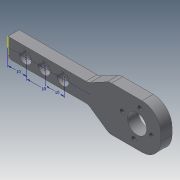
# Autodesk Inventor part: Xmovementarm
Saved by Autodesk Inventor 2019 (Build 230136000, 136)
## iProperties
Created: 2019-01-13
Part Number: Xmovementarm
Material: Aluminum 6061
Document SubType Name: Modeling
Designer: LillaHunden
Density: 2.7 g/cm^3
Appearance: Aluminum - Flat
Mass: 17.0465 g
Surface Area: 40.0048 cm^2
Volume: 6.31351 cm^3
Author: LillaHunden
Autodesk Inventor part; units mm, degrees
ref_plane "YZ Plane" through (0, 0, 0) normal (1, 0, 0) x (0, 1, 0)
ref_plane "XZ Plane" through (0, 0, 0) normal (0, 1, 0) x (-1, 0, 0)
ref_plane "XY Plane" through (0, 0, 0) normal (0, 0, 1) x (1, 0, 0)
sketch "Sketch1" plane through (0, 0, 0) normal (0, 0, 1) x (1, 0, 0)
  line L0 (86.0355, 15.9499) -> (58.5676, 15.9499)
  line L1 (58.5676, 15.9499) -> (58.5676, -7.7845)
  line L2 (58.5676, -7.7845) -> (86.0355, -7.7845)
  line L3 (86.0355, -7.7845) -> (86.0355, 15.9499)
  line L4 (6.25, 0) -> (40, 0) projected
  line L5 (40, 0) -> (40, 10) projected
  line L6 (4.75, 10) -> (40, 10) projected
  line L7 (40, 10) -> (58.5676, 10)
  line L8 (40, 0) -> (58.5676, 0)
  line L9 (58.5676, 15.9499) -> (47.3956, 10)
  line L10 (58.5676, -7.7845) -> (47.3956, 0)
  circle A0 centre (34, 5) radius 2 projected
  line L11 (4.75, 10) -> (4.75, 1.5) projected
  circle A1 centre (14, 5) radius 1.5 projected
  circle A2 centre (34, 5) radius 1.5 projected
  circle A3 centre (24, 5) radius 1.5 projected
  line L12 (6.25, 0) -> (4.75, 1.5) projected
  constraints: 16 end point, 4 point on line, 3 perpendicular, 2 parallel, 1 horizontal
extrude "Extrusion1" add sketch "Sketch1" along normal blind 6 contours L3 L2 L1 L0 | L1 L7 L9 | L1 L8 L5 L7 | L10 L8 L1 | L5 L4 L12 L11 L6 | A0 | A1 | A2 | A3
sketch "Sketch2" plane through (0, 0, 0) normal (0, 0, -1) x (-1, 0, 0)
  circle A0 centre (-73.4131, 4.0423) radius 11 construction
  spline S0 degree 3 poles (-70.2716, -3.9978) (-70.3138, -4.1848) (-70.3928, -4.3613) (-70.5018, -4.5192) (-70.5089, -4.5295) (-70.5162, -4.5398) (-70.5235, -4.5499) (-70.6171, -4.6787) (-70.7297, -4.7921) (-70.8576, -4.8849) (-70.8752, -4.8977) (-70.8931, -4.9101) (-70.9114, -4.9221) (-70.9198, -4.9276) (-70.9284, -4.9331) (-70.9369, -4.9385) (-71.0158, -4.988) (-71.099, -5.0293) (-71.1859, -5.0613) (-71.2374, -5.0803) (-71.2903, -5.096) (-71.3441, -5.1084) (-71.3753, -5.1156) (-71.4068, -5.1217) (-71.4386, -5.1267) (-71.5837, -5.1495) (-71.732, -5.1491) (-71.8775, -5.1259) (-71.8956, -5.123) (-71.9137, -5.1198) (-71.9318, -5.1161) (-71.9426, -5.114) (-71.9535, -5.1117) (-71.9643, -5.1092) (-72.0615, -5.0873) (-72.1559, -5.0551) (-72.2453, -5.0124) (-72.3176, -4.9779) (-72.3864, -4.9368) (-72.4503, -4.8889) (-72.4664, -4.8768) (-72.4822, -4.8643) (-72.4968, -4.8497) knots 0 0 0 0 0.200829 0.200829 0.200829 0.213978 0.213978 0.213978 0.380655 0.380655 0.380655 0.403633 0.403633 0.403633 0.414319 0.414319 0.414319 0.512539 0.512539 0.512539 0.570815 0.570815 0.570815 0.60461 0.60461 0.60461 0.759068 0.759068 0.759068 0.77833 0.77833 0.77833 0.789949 0.789949 0.789949 0.894318 0.894318 0.894318 0.978751 0.978751 0.978751 1 1 1 1 construction
  arc A1 (-73.0396, -4.0484) -> (-72.4967, -4.8495) centre (-71.8011, -3.7936) ccw construction
  spline S1 degree 3 poles (-73.0396, -4.0484) (-73.0842, -3.9099) (-73.1027, -3.7649) (-73.0978, -3.6195) (-73.0972, -3.6016) (-73.0963, -3.5837) (-73.095, -3.5658) (-73.0942, -3.5557) (-73.0934, -3.5457) (-73.0924, -3.5356) (-73.0782, -3.3868) (-73.0398, -3.2412) (-72.9794, -3.105) (-72.9725, -3.0896) (-72.9654, -3.0744) (-72.958, -3.0592) (-72.9531, -3.0492) (-72.9481, -3.0393) (-72.943, -3.0294) (-72.9012, -2.9491) (-72.8517, -2.8734) (-72.7948, -2.8038) (-72.7601, -2.7613) (-72.7225, -2.721) (-72.6825, -2.6829) (-72.6706, -2.6716) (-72.6584, -2.6604) (-72.646, -2.6494) (-72.6345, -2.6393) (-72.6228, -2.6293) (-72.611, -2.6196) (-72.4803, -2.5116) (-72.3306, -2.4274) (-72.1701, -2.3691) (-72.159, -2.365) (-72.1479, -2.3611) (-72.1367, -2.3573) (-72.0422, -2.3254) (-71.945, -2.3027) (-71.8465, -2.2896) (-71.8305, -2.2875) (-71.8144, -2.2856) (-71.7983, -2.284) (-71.7866, -2.2828) (-71.7748, -2.2818) (-71.763, -2.2809) (-71.7023, -2.2762) (-71.6416, -2.2753) (-71.5811, -2.2783) (-71.5527, -2.2796) (-71.5244, -2.2819) (-71.4961, -2.285) (-71.4719, -2.2876) (-71.4478, -2.2909) (-71.424, -2.2973) knots 0 0 0 0 0.153066 0.153066 0.153066 0.171917 0.171917 0.171917 0.182531 0.182531 0.182531 0.339556 0.339556 0.339556 0.35729 0.35729 0.35729 0.369023 0.369023 0.369023 0.464442 0.464442 0.464442 0.522742 0.522742 0.522742 0.540193 0.540193 0.540193 0.556325 0.556325 0.556325 0.734813 0.734813 0.734813 0.747126 0.747126 0.747126 0.851246 0.851246 0.851246 0.868176 0.868176 0.868176 0.880588 0.880588 0.880588 0.944403 0.944403 0.944403 0.974326 0.974326 0.974326 1 1 1 1 construction
  arc A2 (-70.2716, -3.9978) -> (-71.4242, -2.2973) centre (-71.8011, -3.7936) ccw construction
  spline S2 degree 3 poles (-64.0477, 5.4501) (-64.0899, 5.2631) (-64.1689, 5.0866) (-64.2779, 4.9287) (-64.285, 4.9184) (-64.2923, 4.9081) (-64.2996, 4.898) (-64.4061, 4.7515) (-64.5371, 4.6247) (-64.6874, 4.5258) (-64.6959, 4.5203) (-64.7044, 4.5148) (-64.713, 4.5094) (-64.7919, 4.4599) (-64.8751, 4.4186) (-64.962, 4.3866) (-65.0135, 4.3676) (-65.0663, 4.3519) (-65.1202, 4.3395) (-65.1368, 4.3357) (-65.1535, 4.3322) (-65.1703, 4.3289) (-65.185, 4.3261) (-65.1998, 4.3235) (-65.2147, 4.3212) (-65.3598, 4.2984) (-65.5081, 4.2988) (-65.6536, 4.322) (-65.6717, 4.3249) (-65.6898, 4.3282) (-65.7079, 4.3318) (-65.7187, 4.3339) (-65.7296, 4.3362) (-65.7404, 4.3387) (-65.8256, 4.3579) (-65.9086, 4.385) (-65.988, 4.4201) (-65.9992, 4.4251) (-66.0103, 4.4302) (-66.0214, 4.4355) (-66.0678, 4.4576) (-66.1127, 4.4825) (-66.1558, 4.5101) (-66.1799, 4.5256) (-66.2035, 4.5419) (-66.2264, 4.559) (-66.2425, 4.5711) (-66.2583, 4.5836) (-66.2729, 4.5982) knots 0 0 0 0 0.200829 0.200829 0.200829 0.213978 0.213978 0.213978 0.403633 0.403633 0.403633 0.414319 0.414319 0.414319 0.512539 0.512539 0.512539 0.570815 0.570815 0.570815 0.588808 0.588808 0.588808 0.60461 0.60461 0.60461 0.759068 0.759068 0.759068 0.77833 0.77833 0.77833 0.789949 0.789949 0.789949 0.881423 0.881423 0.881423 0.894318 0.894318 0.894318 0.948472 0.948472 0.948472 0.978751 0.978751 0.978751 1 1 1 1 construction
  arc A3 (-66.8157, 5.3996) -> (-66.2728, 4.5984) centre (-65.5772, 5.6543) ccw construction
  spline S3 degree 3 poles (-66.8157, 5.3996) (-66.8603, 5.538) (-66.8788, 5.683) (-66.8739, 5.8284) (-66.8733, 5.8463) (-66.8724, 5.8642) (-66.8711, 5.8821) (-66.8703, 5.8922) (-66.8695, 5.9022) (-66.8685, 5.9123) (-66.8543, 6.0611) (-66.8159, 6.2067) (-66.7555, 6.3429) (-66.7486, 6.3583) (-66.7415, 6.3736) (-66.7341, 6.3887) (-66.7292, 6.3987) (-66.7242, 6.4086) (-66.7191, 6.4185) (-66.6773, 6.4988) (-66.6278, 6.5745) (-66.5709, 6.6441) (-66.5361, 6.6866) (-66.4986, 6.727) (-66.4586, 6.765) (-66.4467, 6.7763) (-66.4345, 6.7875) (-66.4221, 6.7985) (-66.4106, 6.8086) (-66.3989, 6.8186) (-66.3871, 6.8283) (-66.2714, 6.9239) (-66.1407, 7.0009) (-66.0009, 7.0578) (-65.9828, 7.0651) (-65.9646, 7.0722) (-65.9462, 7.0789) (-65.8784, 7.1035) (-65.8088, 7.1234) (-65.7383, 7.1384) (-65.7, 7.1465) (-65.6614, 7.1532) (-65.6226, 7.1583) (-65.6066, 7.1604) (-65.5905, 7.1623) (-65.5744, 7.1639) (-65.5627, 7.1651) (-65.5509, 7.1661) (-65.5391, 7.167) (-65.4784, 7.1717) (-65.4177, 7.1726) (-65.3572, 7.1696) (-65.3288, 7.1683) (-65.3005, 7.166) (-65.2722, 7.163) (-65.248, 7.1603) (-65.2239, 7.157) (-65.2001, 7.1506) knots 0 0 0 0 0.153066 0.153066 0.153066 0.171917 0.171917 0.171917 0.182531 0.182531 0.182531 0.339556 0.339556 0.339556 0.35729 0.35729 0.35729 0.369023 0.369023 0.369023 0.464442 0.464442 0.464442 0.522742 0.522742 0.522742 0.540193 0.540193 0.540193 0.556325 0.556325 0.556325 0.714368 0.714368 0.714368 0.734813 0.734813 0.734813 0.810219 0.810219 0.810219 0.851246 0.851246 0.851246 0.868176 0.868176 0.868176 0.880588 0.880588 0.880588 0.944403 0.944403 0.944403 0.974325 0.974325 0.974325 1 1 1 1 construction
  arc A4 (-64.0477, 5.4501) -> (-65.2003, 7.1506) centre (-65.5772, 5.6543) ccw construction
  spline S4 degree 3 poles (-73.4956, 11.674) (-73.5326, 11.5103) (-73.5978, 11.3546) (-73.6865, 11.2124) (-73.6991, 11.1922) (-73.7122, 11.1723) (-73.7258, 11.1526) (-73.7329, 11.1423) (-73.7402, 11.132) (-73.7476, 11.1219) (-73.8411, 10.9931) (-73.9537, 10.8797) (-74.0816, 10.7869) (-74.0992, 10.7741) (-74.1171, 10.7617) (-74.1354, 10.7497) (-74.1438, 10.7442) (-74.1524, 10.7387) (-74.1609, 10.7333) (-74.2398, 10.6838) (-74.323, 10.6425) (-74.4099, 10.6105) (-74.4614, 10.5915) (-74.5143, 10.5758) (-74.5681, 10.5634) (-74.5847, 10.5596) (-74.6014, 10.5561) (-74.6182, 10.5528) (-74.777, 10.5225) (-74.9412, 10.5203) (-75.1015, 10.5459) (-75.1196, 10.5488) (-75.1377, 10.5521) (-75.1558, 10.5557) (-75.1666, 10.5578) (-75.1775, 10.5602) (-75.1883, 10.5626) (-75.2735, 10.5818) (-75.3565, 10.6089) (-75.4359, 10.644) (-75.4471, 10.649) (-75.4582, 10.6541) (-75.4693, 10.6594) (-75.5416, 10.6939) (-75.6104, 10.735) (-75.6743, 10.7829) (-75.6904, 10.795) (-75.7062, 10.8075) (-75.7208, 10.8221) knots 0 0 0 0 0.175859 0.175859 0.175859 0.200829 0.200829 0.200829 0.213978 0.213978 0.213978 0.380655 0.380655 0.380655 0.403633 0.403633 0.403633 0.414319 0.414319 0.414319 0.512539 0.512539 0.512539 0.570815 0.570815 0.570815 0.588808 0.588808 0.588808 0.759068 0.759068 0.759068 0.77833 0.77833 0.77833 0.789949 0.789949 0.789949 0.881423 0.881423 0.881423 0.894318 0.894318 0.894318 0.978751 0.978751 0.978751 1 1 1 1 construction
  arc A5 (-76.2636, 11.6235) -> (-75.7207, 10.8223) centre (-75.0251, 11.8783) ccw construction
  spline S5 degree 3 poles (-76.2636, 11.6235) (-76.3168, 11.7886) (-76.333, 11.9632) (-76.3164, 12.1362) (-76.3022, 12.285) (-76.2638, 12.4306) (-76.2034, 12.5668) (-76.1965, 12.5822) (-76.1894, 12.5975) (-76.182, 12.6126) (-76.1771, 12.6226) (-76.1721, 12.6326) (-76.167, 12.6424) (-76.1252, 12.7227) (-76.0757, 12.7984) (-76.0188, 12.868) (-75.9841, 12.9106) (-75.9465, 12.9509) (-75.9065, 12.9889) (-75.8946, 13.0002) (-75.8824, 13.0114) (-75.87, 13.0224) (-75.8585, 13.0325) (-75.8468, 13.0425) (-75.835, 13.0522) (-75.7193, 13.1478) (-75.5886, 13.2248) (-75.4488, 13.2817) (-75.4307, 13.289) (-75.4125, 13.2961) (-75.3941, 13.3028) (-75.383, 13.3068) (-75.3719, 13.3107) (-75.3607, 13.3145) (-75.2662, 13.3464) (-75.169, 13.3691) (-75.0705, 13.3822) (-75.0545, 13.3844) (-75.0384, 13.3862) (-75.0224, 13.3878) (-75.0106, 13.389) (-74.9988, 13.3901) (-74.987, 13.391) (-74.8979, 13.3978) (-74.8086, 13.3965) (-74.7201, 13.3869) (-74.6959, 13.3842) (-74.6718, 13.3809) (-74.648, 13.3745) knots 0 0 0 0 0.182531 0.182531 0.182531 0.339556 0.339556 0.339556 0.357289 0.357289 0.357289 0.369023 0.369023 0.369023 0.464442 0.464442 0.464442 0.522742 0.522742 0.522742 0.540193 0.540193 0.540193 0.556325 0.556325 0.556325 0.714368 0.714368 0.714368 0.734813 0.734813 0.734813 0.747125 0.747125 0.747125 0.851246 0.851246 0.851246 0.868176 0.868176 0.868176 0.880588 0.880588 0.880588 0.974325 0.974325 0.974325 1 1 1 1 construction
  arc A6 (-73.4956, 11.674) -> (-74.6482, 13.3745) centre (-75.0251, 11.8783) ccw construction
  spline S6 degree 3 poles (-79.7195, 2.2261) (-79.7995, 1.8717) (-80.0134, 1.5509) (-80.3055, 1.339) (-80.3231, 1.3262) (-80.3411, 1.3138) (-80.3593, 1.3018) (-80.3677, 1.2963) (-80.3763, 1.2908) (-80.3848, 1.2854) (-80.4637, 1.2359) (-80.5469, 1.1946) (-80.6338, 1.1626) (-80.6853, 1.1436) (-80.7382, 1.1279) (-80.792, 1.1155) (-80.8086, 1.1117) (-80.8253, 1.1081) (-80.8421, 1.1049) (-80.8568, 1.1021) (-80.8716, 1.0995) (-80.8865, 1.0972) (-81.0316, 1.0744) (-81.18, 1.0748) (-81.3254, 1.098) (-81.3435, 1.1009) (-81.3616, 1.1041) (-81.3797, 1.1078) (-81.3905, 1.1099) (-81.4014, 1.1122) (-81.4122, 1.1147) (-81.4974, 1.1339) (-81.5804, 1.161) (-81.6598, 1.1961) (-81.671, 1.2011) (-81.6821, 1.2062) (-81.6932, 1.2115) (-81.7655, 1.246) (-81.8343, 1.2871) (-81.8982, 1.335) (-81.9143, 1.3471) (-81.9301, 1.3596) (-81.9447, 1.3742) knots 0 0 0 0 0.380655 0.380655 0.380655 0.403633 0.403633 0.403633 0.414319 0.414319 0.414319 0.512539 0.512539 0.512539 0.570815 0.570815 0.570815 0.588808 0.588808 0.588808 0.60461 0.60461 0.60461 0.759068 0.759068 0.759068 0.77833 0.77833 0.77833 0.789949 0.789949 0.789949 0.881423 0.881423 0.881423 0.894318 0.894318 0.894318 0.978751 0.978751 0.978751 1 1 1 1 construction
  arc A7 (-82.4875, 2.1755) -> (-81.9446, 1.3744) centre (-81.249, 2.4303) ccw construction
  spline S7 degree 3 poles (-82.4875, 2.1755) (-82.5321, 2.314) (-82.5506, 2.459) (-82.5457, 2.6044) (-82.5451, 2.6223) (-82.5442, 2.6402) (-82.5429, 2.6581) (-82.5421, 2.6682) (-82.5413, 2.6782) (-82.5403, 2.6883) (-82.5245, 2.8539) (-82.4788, 3.0156) (-82.4059, 3.1647) (-82.401, 3.1747) (-82.396, 3.1846) (-82.3909, 3.1945) (-82.3491, 3.2748) (-82.2996, 3.3505) (-82.2427, 3.4201) (-82.208, 3.4626) (-82.1704, 3.503) (-82.1304, 3.541) (-82.1185, 3.5523) (-82.1063, 3.5635) (-82.0939, 3.5745) (-82.0824, 3.5846) (-82.0707, 3.5946) (-82.0589, 3.6043) (-81.9282, 3.7123) (-81.7785, 3.7965) (-81.618, 3.8549) (-81.6069, 3.8589) (-81.5958, 3.8628) (-81.5846, 3.8666) (-81.4748, 3.9037) (-81.3612, 3.9284) (-81.2463, 3.9399) (-81.2345, 3.9411) (-81.2227, 3.9421) (-81.2109, 3.943) (-81.1502, 3.9477) (-81.0895, 3.9486) (-81.029, 3.9456) (-81.0006, 3.9443) (-80.9723, 3.942) (-80.944, 3.939) (-80.9198, 3.9363) (-80.8957, 3.933) (-80.8719, 3.9266) knots 0 0 0 0 0.153066 0.153066 0.153066 0.171917 0.171917 0.171917 0.182531 0.182531 0.182531 0.357289 0.357289 0.357289 0.369023 0.369023 0.369023 0.464442 0.464442 0.464442 0.522742 0.522742 0.522742 0.540193 0.540193 0.540193 0.556325 0.556325 0.556325 0.734813 0.734813 0.734813 0.747125 0.747125 0.747125 0.868176 0.868176 0.868176 0.880588 0.880588 0.880588 0.944403 0.944403 0.944403 0.974325 0.974325 0.974325 1 1 1 1 construction
  arc A8 (-79.7195, 2.2261) -> (-80.8721, 3.9266) centre (-81.249, 2.4303) ccw construction
  circle A9 centre (-73.4131, 4.0423) radius 5.15 construction
  point P0 (0, 0)
  constraints: 4 coincident
hole "Hole1" at (81.249, 2.4303, 0) at (75.0251, 11.8783, 0) at (65.5772, 5.6543, 0) at (71.8011, -3.7936, 0) direction (0, 0, 1) diameter 2.459 depth 8.8 thread size "M3x0.5" class "6H" standard "ISO Metric profile"
sketch "Sketch3" plane through (0, 0, 6) normal (0, 0, 1) x (1, 0, 0)
  circle A0 centre (73.4131, 4.0423) radius 11
  spline S0 degree 3 poles (70.2716, -3.9978) (70.3138, -4.1848) (70.3928, -4.3613) (70.5018, -4.5192) (70.5089, -4.5295) (70.5162, -4.5398) (70.5235, -4.5499) (70.6171, -4.6787) (70.7297, -4.7921) (70.8576, -4.8849) (70.8752, -4.8977) (70.8931, -4.9101) (70.9114, -4.9221) (70.9198, -4.9276) (70.9284, -4.9331) (70.9369, -4.9385) (71.0158, -4.988) (71.099, -5.0293) (71.1859, -5.0613) (71.2374, -5.0803) (71.2903, -5.096) (71.3441, -5.1084) (71.3753, -5.1156) (71.4068, -5.1217) (71.4386, -5.1267) (71.5837, -5.1495) (71.732, -5.1491) (71.8775, -5.1259) (71.8956, -5.123) (71.9137, -5.1198) (71.9318, -5.1161) (71.9426, -5.114) (71.9535, -5.1117) (71.9643, -5.1092) (72.0615, -5.0873) (72.1559, -5.0551) (72.2453, -5.0124) (72.3176, -4.9779) (72.3864, -4.9368) (72.4503, -4.8889) (72.4664, -4.8768) (72.4822, -4.8643) (72.4968, -4.8497) knots 0 0 0 0 0.200829 0.200829 0.200829 0.213978 0.213978 0.213978 0.380655 0.380655 0.380655 0.403633 0.403633 0.403633 0.414319 0.414319 0.414319 0.512539 0.512539 0.512539 0.570815 0.570815 0.570815 0.60461 0.60461 0.60461 0.759068 0.759068 0.759068 0.77833 0.77833 0.77833 0.789949 0.789949 0.789949 0.894318 0.894318 0.894318 0.978751 0.978751 0.978751 1 1 1 1
  arc A1 (72.4967, -4.8495) -> (73.0396, -4.0484) centre (71.8011, -3.7936) ccw
  spline S1 degree 3 poles (73.0396, -4.0484) (73.0842, -3.9099) (73.1027, -3.7649) (73.0978, -3.6195) (73.0972, -3.6016) (73.0963, -3.5837) (73.095, -3.5658) (73.0942, -3.5557) (73.0934, -3.5457) (73.0924, -3.5356) (73.0782, -3.3868) (73.0398, -3.2412) (72.9794, -3.105) (72.9725, -3.0896) (72.9654, -3.0744) (72.958, -3.0592) (72.9531, -3.0492) (72.9481, -3.0393) (72.943, -3.0294) (72.9012, -2.9491) (72.8517, -2.8734) (72.7948, -2.8038) (72.7601, -2.7613) (72.7225, -2.721) (72.6825, -2.6829) (72.6706, -2.6716) (72.6584, -2.6604) (72.646, -2.6494) (72.6345, -2.6393) (72.6228, -2.6293) (72.611, -2.6196) (72.4803, -2.5116) (72.3306, -2.4274) (72.1701, -2.3691) (72.159, -2.365) (72.1479, -2.3611) (72.1367, -2.3573) (72.0422, -2.3254) (71.945, -2.3027) (71.8465, -2.2896) (71.8305, -2.2875) (71.8144, -2.2856) (71.7983, -2.284) (71.7866, -2.2828) (71.7748, -2.2818) (71.763, -2.2809) (71.7023, -2.2762) (71.6416, -2.2753) (71.5811, -2.2783) (71.5527, -2.2796) (71.5244, -2.2819) (71.4961, -2.285) (71.4719, -2.2876) (71.4478, -2.2909) (71.424, -2.2973) knots 0 0 0 0 0.153066 0.153066 0.153066 0.171917 0.171917 0.171917 0.182531 0.182531 0.182531 0.339556 0.339556 0.339556 0.35729 0.35729 0.35729 0.369023 0.369023 0.369023 0.464442 0.464442 0.464442 0.522742 0.522742 0.522742 0.540193 0.540193 0.540193 0.556325 0.556325 0.556325 0.734813 0.734813 0.734813 0.747126 0.747126 0.747126 0.851246 0.851246 0.851246 0.868176 0.868176 0.868176 0.880588 0.880588 0.880588 0.944403 0.944403 0.944403 0.974326 0.974326 0.974326 1 1 1 1
  arc A2 (71.4242, -2.2973) -> (70.2716, -3.9978) centre (71.8011, -3.7936) ccw
  spline S2 degree 3 poles (64.0477, 5.4501) (64.0899, 5.2631) (64.1689, 5.0866) (64.2779, 4.9287) (64.285, 4.9184) (64.2923, 4.9081) (64.2996, 4.898) (64.4061, 4.7515) (64.5371, 4.6247) (64.6874, 4.5258) (64.6959, 4.5203) (64.7044, 4.5148) (64.713, 4.5094) (64.7919, 4.4599) (64.8751, 4.4186) (64.962, 4.3866) (65.0135, 4.3676) (65.0663, 4.3519) (65.1202, 4.3395) (65.1368, 4.3357) (65.1535, 4.3322) (65.1703, 4.3289) (65.185, 4.3261) (65.1998, 4.3235) (65.2147, 4.3212) (65.3598, 4.2984) (65.5081, 4.2988) (65.6536, 4.322) (65.6717, 4.3249) (65.6898, 4.3282) (65.7079, 4.3318) (65.7187, 4.3339) (65.7296, 4.3362) (65.7404, 4.3387) (65.8256, 4.3579) (65.9086, 4.385) (65.988, 4.4201) (65.9992, 4.4251) (66.0103, 4.4302) (66.0214, 4.4355) (66.0678, 4.4576) (66.1127, 4.4825) (66.1558, 4.5101) (66.1799, 4.5256) (66.2035, 4.5419) (66.2264, 4.559) (66.2425, 4.5711) (66.2583, 4.5836) (66.2729, 4.5982) knots 0 0 0 0 0.200829 0.200829 0.200829 0.213978 0.213978 0.213978 0.403633 0.403633 0.403633 0.414319 0.414319 0.414319 0.512539 0.512539 0.512539 0.570815 0.570815 0.570815 0.588808 0.588808 0.588808 0.60461 0.60461 0.60461 0.759068 0.759068 0.759068 0.77833 0.77833 0.77833 0.789949 0.789949 0.789949 0.881423 0.881423 0.881423 0.894318 0.894318 0.894318 0.948472 0.948472 0.948472 0.978751 0.978751 0.978751 1 1 1 1
  arc A3 (66.2728, 4.5984) -> (66.8157, 5.3996) centre (65.5772, 5.6543) ccw
  spline S3 degree 3 poles (66.8157, 5.3996) (66.8603, 5.538) (66.8788, 5.683) (66.8739, 5.8284) (66.8733, 5.8463) (66.8724, 5.8642) (66.8711, 5.8821) (66.8703, 5.8922) (66.8695, 5.9022) (66.8685, 5.9123) (66.8543, 6.0611) (66.8159, 6.2067) (66.7555, 6.3429) (66.7486, 6.3583) (66.7415, 6.3736) (66.7341, 6.3887) (66.7292, 6.3987) (66.7242, 6.4086) (66.7191, 6.4185) (66.6773, 6.4988) (66.6278, 6.5745) (66.5709, 6.6441) (66.5361, 6.6866) (66.4986, 6.727) (66.4586, 6.765) (66.4467, 6.7763) (66.4345, 6.7875) (66.4221, 6.7985) (66.4106, 6.8086) (66.3989, 6.8186) (66.3871, 6.8283) (66.2714, 6.9239) (66.1407, 7.0009) (66.0009, 7.0578) (65.9828, 7.0651) (65.9646, 7.0722) (65.9462, 7.0789) (65.8784, 7.1035) (65.8088, 7.1234) (65.7383, 7.1384) (65.7, 7.1465) (65.6614, 7.1532) (65.6226, 7.1583) (65.6066, 7.1604) (65.5905, 7.1623) (65.5744, 7.1639) (65.5627, 7.1651) (65.5509, 7.1661) (65.5391, 7.167) (65.4784, 7.1717) (65.4177, 7.1726) (65.3572, 7.1696) (65.3288, 7.1683) (65.3005, 7.166) (65.2722, 7.163) (65.248, 7.1603) (65.2239, 7.157) (65.2001, 7.1506) knots 0 0 0 0 0.153066 0.153066 0.153066 0.171917 0.171917 0.171917 0.182531 0.182531 0.182531 0.339556 0.339556 0.339556 0.35729 0.35729 0.35729 0.369023 0.369023 0.369023 0.464442 0.464442 0.464442 0.522742 0.522742 0.522742 0.540193 0.540193 0.540193 0.556325 0.556325 0.556325 0.714368 0.714368 0.714368 0.734813 0.734813 0.734813 0.810219 0.810219 0.810219 0.851246 0.851246 0.851246 0.868176 0.868176 0.868176 0.880588 0.880588 0.880588 0.944403 0.944403 0.944403 0.974325 0.974325 0.974325 1 1 1 1
  arc A4 (65.2003, 7.1506) -> (64.0477, 5.4501) centre (65.5772, 5.6543) ccw
  spline S4 degree 3 poles (73.4956, 11.674) (73.5326, 11.5103) (73.5978, 11.3546) (73.6865, 11.2124) (73.6991, 11.1922) (73.7122, 11.1723) (73.7258, 11.1526) (73.7329, 11.1423) (73.7402, 11.132) (73.7476, 11.1219) (73.8411, 10.9931) (73.9537, 10.8797) (74.0816, 10.7869) (74.0992, 10.7741) (74.1171, 10.7617) (74.1354, 10.7497) (74.1438, 10.7442) (74.1524, 10.7387) (74.1609, 10.7333) (74.2398, 10.6838) (74.323, 10.6425) (74.4099, 10.6105) (74.4614, 10.5915) (74.5143, 10.5758) (74.5681, 10.5634) (74.5847, 10.5596) (74.6014, 10.5561) (74.6182, 10.5528) (74.777, 10.5225) (74.9412, 10.5203) (75.1015, 10.5459) (75.1196, 10.5488) (75.1377, 10.5521) (75.1558, 10.5557) (75.1666, 10.5578) (75.1775, 10.5602) (75.1883, 10.5626) (75.2735, 10.5818) (75.3565, 10.6089) (75.4359, 10.644) (75.4471, 10.649) (75.4582, 10.6541) (75.4693, 10.6594) (75.5416, 10.6939) (75.6104, 10.735) (75.6743, 10.7829) (75.6904, 10.795) (75.7062, 10.8075) (75.7208, 10.8221) knots 0 0 0 0 0.175859 0.175859 0.175859 0.200829 0.200829 0.200829 0.213978 0.213978 0.213978 0.380655 0.380655 0.380655 0.403633 0.403633 0.403633 0.414319 0.414319 0.414319 0.512539 0.512539 0.512539 0.570815 0.570815 0.570815 0.588808 0.588808 0.588808 0.759068 0.759068 0.759068 0.77833 0.77833 0.77833 0.789949 0.789949 0.789949 0.881423 0.881423 0.881423 0.894318 0.894318 0.894318 0.978751 0.978751 0.978751 1 1 1 1
  arc A5 (75.7207, 10.8223) -> (76.2636, 11.6235) centre (75.0251, 11.8783) ccw
  spline S5 degree 3 poles (76.2636, 11.6235) (76.3168, 11.7886) (76.333, 11.9632) (76.3164, 12.1362) (76.3022, 12.285) (76.2638, 12.4306) (76.2034, 12.5668) (76.1965, 12.5822) (76.1894, 12.5975) (76.182, 12.6126) (76.1771, 12.6226) (76.1721, 12.6326) (76.167, 12.6424) (76.1252, 12.7227) (76.0757, 12.7984) (76.0188, 12.868) (75.9841, 12.9106) (75.9465, 12.9509) (75.9065, 12.9889) (75.8946, 13.0002) (75.8824, 13.0114) (75.87, 13.0224) (75.8585, 13.0325) (75.8468, 13.0425) (75.835, 13.0522) (75.7193, 13.1478) (75.5886, 13.2248) (75.4488, 13.2817) (75.4307, 13.289) (75.4125, 13.2961) (75.3941, 13.3028) (75.383, 13.3068) (75.3719, 13.3107) (75.3607, 13.3145) (75.2662, 13.3464) (75.169, 13.3691) (75.0705, 13.3822) (75.0545, 13.3844) (75.0384, 13.3862) (75.0224, 13.3878) (75.0106, 13.389) (74.9988, 13.3901) (74.987, 13.391) (74.8979, 13.3978) (74.8086, 13.3965) (74.7201, 13.3869) (74.6959, 13.3842) (74.6718, 13.3809) (74.648, 13.3745) knots 0 0 0 0 0.182531 0.182531 0.182531 0.339556 0.339556 0.339556 0.357289 0.357289 0.357289 0.369023 0.369023 0.369023 0.464442 0.464442 0.464442 0.522742 0.522742 0.522742 0.540193 0.540193 0.540193 0.556325 0.556325 0.556325 0.714368 0.714368 0.714368 0.734813 0.734813 0.734813 0.747125 0.747125 0.747125 0.851246 0.851246 0.851246 0.868176 0.868176 0.868176 0.880588 0.880588 0.880588 0.974325 0.974325 0.974325 1 1 1 1
  arc A6 (74.6482, 13.3745) -> (73.4956, 11.674) centre (75.0251, 11.8783) ccw
  spline S6 degree 3 poles (79.7195, 2.2261) (79.7995, 1.8717) (80.0134, 1.5509) (80.3055, 1.339) (80.3231, 1.3262) (80.3411, 1.3138) (80.3593, 1.3018) (80.3677, 1.2963) (80.3763, 1.2908) (80.3848, 1.2854) (80.4637, 1.2359) (80.5469, 1.1946) (80.6338, 1.1626) (80.6853, 1.1436) (80.7382, 1.1279) (80.792, 1.1155) (80.8086, 1.1117) (80.8253, 1.1081) (80.8421, 1.1049) (80.8568, 1.1021) (80.8716, 1.0995) (80.8865, 1.0972) (81.0316, 1.0744) (81.18, 1.0748) (81.3254, 1.098) (81.3435, 1.1009) (81.3616, 1.1041) (81.3797, 1.1078) (81.3905, 1.1099) (81.4014, 1.1122) (81.4122, 1.1147) (81.4974, 1.1339) (81.5804, 1.161) (81.6598, 1.1961) (81.671, 1.2011) (81.6821, 1.2062) (81.6932, 1.2115) (81.7655, 1.246) (81.8343, 1.2871) (81.8982, 1.335) (81.9143, 1.3471) (81.9301, 1.3596) (81.9447, 1.3742) knots 0 0 0 0 0.380655 0.380655 0.380655 0.403633 0.403633 0.403633 0.414319 0.414319 0.414319 0.512539 0.512539 0.512539 0.570815 0.570815 0.570815 0.588808 0.588808 0.588808 0.60461 0.60461 0.60461 0.759068 0.759068 0.759068 0.77833 0.77833 0.77833 0.789949 0.789949 0.789949 0.881423 0.881423 0.881423 0.894318 0.894318 0.894318 0.978751 0.978751 0.978751 1 1 1 1
  arc A7 (81.9446, 1.3744) -> (82.4875, 2.1755) centre (81.249, 2.4303) ccw
  spline S7 degree 3 poles (82.4875, 2.1755) (82.5321, 2.314) (82.5506, 2.459) (82.5457, 2.6044) (82.5451, 2.6223) (82.5442, 2.6402) (82.5429, 2.6581) (82.5421, 2.6682) (82.5413, 2.6782) (82.5403, 2.6883) (82.5245, 2.8539) (82.4788, 3.0156) (82.4059, 3.1647) (82.401, 3.1747) (82.396, 3.1846) (82.3909, 3.1945) (82.3491, 3.2748) (82.2996, 3.3505) (82.2427, 3.4201) (82.208, 3.4626) (82.1704, 3.503) (82.1304, 3.541) (82.1185, 3.5523) (82.1063, 3.5635) (82.0939, 3.5745) (82.0824, 3.5846) (82.0707, 3.5946) (82.0589, 3.6043) (81.9282, 3.7123) (81.7785, 3.7965) (81.618, 3.8549) (81.6069, 3.8589) (81.5958, 3.8628) (81.5846, 3.8666) (81.4748, 3.9037) (81.3612, 3.9284) (81.2463, 3.9399) (81.2345, 3.9411) (81.2227, 3.9421) (81.2109, 3.943) (81.1502, 3.9477) (81.0895, 3.9486) (81.029, 3.9456) (81.0006, 3.9443) (80.9723, 3.942) (80.944, 3.939) (80.9198, 3.9363) (80.8957, 3.933) (80.8719, 3.9266) knots 0 0 0 0 0.153066 0.153066 0.153066 0.171917 0.171917 0.171917 0.182531 0.182531 0.182531 0.357289 0.357289 0.357289 0.369023 0.369023 0.369023 0.464442 0.464442 0.464442 0.522742 0.522742 0.522742 0.540193 0.540193 0.540193 0.556325 0.556325 0.556325 0.734813 0.734813 0.734813 0.747125 0.747125 0.747125 0.868176 0.868176 0.868176 0.880588 0.880588 0.880588 0.944403 0.944403 0.944403 0.974325 0.974325 0.974325 1 1 1 1
  arc A8 (80.8721, 3.9266) -> (79.7195, 2.2261) centre (81.249, 2.4303) ccw
  circle A9 centre (73.4131, 4.0423) radius 5.15
  point P0 (0, 0)
extrude "Extrusion2" cut sketch "Sketch3" against normal through all contours A9
sketch "Sketch4" plane through (0, 0, 6) normal (0, 0, 1) x (1, 0, 0)
  line L0 (4.75, 10) -> (4.75, 1.5) projected
  line L1 (4.75, 5) -> (48.7838, 5) construction
  point P0 (4.75, 0)
  point P1 (14.75, 5)
  point P2 (24.75, 5)
  point P3 (34.75, 5)
  dimension "d38" = 10
  dimension "d39" = 10
  dimension "d40" = 10
  constraints: 4 point on line, 2 end point, 1 horizontal
  measures "d38" distance of point (14.75, 5) L1.start
  measures "d39" distance of point (24.75, 5) point (14.75, 5)
  measures "d40" distance of point (34.75, 5) point (24.75, 5)
sketch "Sketch7" plane through (0, 0, 6) normal (0, 0, 1) x (1, 0, 0)
  point P0 (14, 5)
  point P1 (24, 5)
  point P2 (34, 5)
sketch "Sketch8" plane through (0, 0, 6) normal (0, 0, 1) x (1, 0, 0)
  point P0 (34, 5)
  point P1 (14, 5)
  point P2 (24, 5)
hole "Hole5" at (34, 5, 6) at (14, 5, 6) at (24, 5, 6) direction (0, 0, -1) diameter 3.4 depth 6 counterbore diameter 6.5 counterbore depth 3.4
fillet "Fillet1" radius 5 4 edges at (47.3956, 0, 3) (47.3956, 10, 3) (58.5676, -7.7845, 3) (58.5676, 15.9499, 3)
fillet "Fillet2" radius 10 2 edges at (86.0355, -7.7845, 3) (86.0355, 15.9499, 3)
equation "\"d13\" = d11"
equation "\"d11\" = 14"
body "Solid1"
